Autodesk Inventor part; units mm, degrees
(part 3 of 3)
  spline S409 degree 2 poles (72.0814, -54.0962) (72.3533, -53.7947) (73.1591, -53.4733) (73.6237, -53.4733) knots 0 0 0 1 2 2 2
  spline S410 degree 2 poles (73.6237, -53.4733) (73.9994, -53.4733) (74.7014, -53.6859) (74.9733, -53.8243) knots 0 0 0 1 2 2 2
  line L406 (74.9733, -53.8243) -> (74.9733, -54.6894)
  line L407 (74.9733, -54.6894) -> (74.9288, -54.6894)
  spline S411 degree 2 poles (74.9288, -54.6894) (74.8447, -54.6202) (74.5877, -54.4422) (74.4048, -54.3483) knots 0 0 0 1 2 2 2
  spline S412 degree 2 poles (74.4048, -54.3483) (74.2417, -54.2692) (73.8066, -54.1456) (73.6089, -54.1456) knots 0 0 0 1 2 2 2
  spline S413 degree 2 poles (73.6089, -54.1456) (73.0108, -54.1456) (72.2841, -55.0503) (72.2841, -55.8758) knots 0 0 0 1 2 2 2
  spline S414 degree 2 poles (72.2841, -55.8758) (72.2841, -56.6815) (72.9861, -57.5862) (73.6089, -57.5862) knots 0 0 0 1 2 2 2
  spline S415 degree 2 poles (73.6089, -57.5862) (73.9846, -57.5862) (74.6668, -57.2747) (74.9288, -57.0325) knots 0 0 0 1 2 2 2
  line L408 (74.9288, -57.0325) -> (74.9733, -57.0325)
  line L409 (74.9733, -57.0325) -> (74.9733, -57.8976)
  spline S416 degree 2 poles (74.9733, -57.8976) (74.8596, -57.952) (74.5135, -58.1052) (74.3751, -58.1398) knots 0 0 0 1 2 2 2
  spline S417 degree 2 poles (74.3751, -58.1398) (74.1774, -58.1991) (73.866, -58.2584) (73.6237, -58.2584) knots 0 0 0 1 2 2 2
  line L410 (76.4612, -58.1546) -> (75.69, -58.1546)
  line L411 (75.69, -58.1546) -> (75.69, -53.5772)
  line L412 (75.69, -53.5772) -> (76.4612, -53.5772)
  line L413 (76.4612, -53.5772) -> (76.4612, -58.1546)
  line L414 (76.5156, -52.8159) -> (75.6406, -52.8159)
  line L415 (75.6406, -52.8159) -> (75.6406, -52.0151)
  line L416 (75.6406, -52.0151) -> (76.5156, -52.0151)
  line L417 (76.5156, -52.0151) -> (76.5156, -52.8159)
  line L418 (-27.0263, -68.1981) -> (-27.0263, -62.8198)
  line L419 (-27.0263, -62.8198) -> (-29.0728, -62.8198)
  line L420 (-29.0728, -62.8198) -> (-29.0728, -62.0981)
  line L421 (-29.0728, -62.0981) -> (-24.169, -62.0981)
  line L422 (-24.169, -62.0981) -> (-24.169, -62.8198)
  line L423 (-24.169, -62.8198) -> (-26.2156, -62.8198)
  line L424 (-26.2156, -62.8198) -> (-26.2156, -68.1981)
  line L425 (-26.2156, -68.1981) -> (-27.0263, -68.1981)
  line L426 (-21.1833, -64.4462) -> (-21.2229, -64.4462)
  spline S418 degree 2 poles (-21.2229, -64.4462) (-21.3118, -64.4215) (-21.5046, -64.4116) (-21.6381, -64.4116) knots 0 0 0 1 2 2 2
  spline S419 degree 2 poles (-21.6381, -64.4116) (-21.9495, -64.4116) (-22.5625, -64.6834) (-22.8393, -64.9504) knots 0 0 0 1 2 2 2
  line L427 (-22.8393, -64.9504) -> (-22.8393, -68.1981)
  line L428 (-22.8393, -68.1981) -> (-23.6105, -68.1981)
  line L429 (-23.6105, -68.1981) -> (-23.6105, -63.6206)
  line L430 (-23.6105, -63.6206) -> (-22.8393, -63.6206)
  line L431 (-22.8393, -63.6206) -> (-22.8393, -64.3028)
  spline S420 degree 2 poles (-22.8393, -64.3028) (-22.4191, -63.9271) (-21.7913, -63.6206) (-21.4947, -63.6206) knots 0 0 0 1 2 2 2
  spline S421 degree 2 poles (-21.4947, -63.6206) (-21.3761, -63.6206) (-21.2575, -63.6305) (-21.1833, -63.6454) knots 0 0 0 1 2 2 2
  line L432 (-21.1833, -63.6454) -> (-21.1833, -64.4462)
  line L433 (-19.7992, -68.1981) -> (-20.5703, -68.1981)
  line L434 (-20.5703, -68.1981) -> (-20.5703, -63.6206)
  line L435 (-20.5703, -63.6206) -> (-19.7992, -63.6206)
  line L436 (-19.7992, -63.6206) -> (-19.7992, -68.1981)
  line L437 (-19.7448, -62.8594) -> (-20.6198, -62.8594)
  line L438 (-20.6198, -62.8594) -> (-20.6198, -62.0586)
  line L439 (-20.6198, -62.0586) -> (-19.7448, -62.0586)
  line L440 (-19.7448, -62.0586) -> (-19.7448, -62.8594)
  spline S422 degree 2 poles (-16.68, -68.3019) (-17.7774, -68.3019) (-18.9836, -67.0711) (-18.9836, -65.9341) knots 0 0 0 1 2 2 2
  spline S423 degree 2 poles (-18.9836, -65.9341) (-18.9836, -64.8169) (-17.812, -63.4921) (-16.8678, -63.4921) knots 0 0 0 1 2 2 2
  spline S424 degree 2 poles (-16.8678, -63.4921) (-16.4427, -63.4921) (-15.7853, -63.7393) (-15.543, -64.0013) knots 0 0 0 1 2 2 2
  spline S425 degree 2 poles (-15.543, -64.0013) (-15.2959, -64.2633) (-15.0339, -65.0196) (-15.0339, -65.5683) knots 0 0 0 1 2 2 2
  line L441 (-15.0339, -65.5683) -> (-15.0339, -65.9885)
  line L442 (-15.0339, -65.9885) -> (-18.2025, -65.9885)
  spline S426 degree 2 poles (-18.2025, -65.9885) (-18.2025, -66.7843) (-17.4017, -67.6296) (-16.6899, -67.6296) knots 0 0 0 1 2 2 2
  spline S427 degree 2 poles (-16.6899, -67.6296) (-16.4378, -67.6296) (-15.9484, -67.5159) (-15.7507, -67.427) knots 0 0 0 1 2 2 2
  spline S428 degree 2 poles (-15.7507, -67.427) (-15.543, -67.3281) (-15.2563, -67.1551) (-15.1624, -67.076) knots 0 0 0 1 2 2 2
  line L443 (-15.1624, -67.076) -> (-15.1179, -67.076)
  line L444 (-15.1179, -67.076) -> (-15.1179, -67.9164)
  spline S429 degree 2 poles (-15.1179, -67.9164) (-15.2514, -67.9707) (-15.6567, -68.1289) (-15.8149, -68.1734) knots 0 0 0 1 2 2 2
  spline S430 degree 2 poles (-15.8149, -68.1734) (-16.0374, -68.2377) (-16.4032, -68.3019) (-16.68, -68.3019) knots 0 0 0 1 2 2 2
  spline S431 degree 2 poles (-15.7853, -65.4002) (-15.7951, -65.0888) (-15.9237, -64.634) (-16.0472, -64.4808) knots 0 0 0 1 2 2 2
  spline S432 degree 2 poles (-16.0472, -64.4808) (-16.1807, -64.3078) (-16.6009, -64.1249) (-16.9123, -64.1249) knots 0 0 0 1 2 2 2
  spline S433 degree 2 poles (-16.9123, -64.1249) (-17.2188, -64.1249) (-17.6489, -64.3078) (-17.8268, -64.4857) knots 0 0 0 1 2 2 2
  spline S434 degree 2 poles (-17.8268, -64.4857) (-17.9998, -64.6686) (-18.1778, -65.1086) (-18.2025, -65.4002) knots 0 0 0 1 2 2 2
  line L445 (-18.2025, -65.4002) -> (-15.7853, -65.4002)
  line L446 (-10.6591, -68.1981) -> (-11.4302, -68.1981)
  line L447 (-11.4302, -68.1981) -> (-11.4302, -65.5881)
  spline S435 degree 2 poles (-11.4302, -65.5881) (-11.4302, -65.2717) (-11.4895, -64.7279) (-11.5785, -64.5648) knots 0 0 0 1 2 2 2
  spline S436 degree 2 poles (-11.5785, -64.5648) (-11.6724, -64.3918) (-12.0086, -64.2237) (-12.2953, -64.2237) knots 0 0 0 1 2 2 2
  spline S437 degree 2 poles (-12.2953, -64.2237) (-12.582, -64.2237) (-13.19, -64.5302) (-13.4817, -64.7774) knots 0 0 0 1 2 2 2
  line L448 (-13.4817, -64.7774) -> (-13.4817, -68.1981)
  line L449 (-13.4817, -68.1981) -> (-14.2528, -68.1981)
  line L450 (-14.2528, -68.1981) -> (-14.2528, -63.6206)
  line L451 (-14.2528, -63.6206) -> (-13.4817, -63.6206)
  line L452 (-13.4817, -63.6206) -> (-13.4817, -64.1298)
  spline S438 degree 2 poles (-13.4817, -64.1298) (-13.1357, -63.8184) (-12.4683, -63.4921) (-12.0926, -63.4921) knots 0 0 0 1 2 2 2
  spline S439 degree 2 poles (-12.0926, -63.4921) (-11.4203, -63.4921) (-10.6591, -64.3819) (-10.6591, -65.2272) knots 0 0 0 1 2 2 2
  line L453 (-10.6591, -65.2272) -> (-10.6591, -68.1981)
  line L454 (-5.9827, -68.1981) -> (-6.7539, -68.1981)
  line L455 (-6.7539, -68.1981) -> (-6.7539, -65.5881)
  spline S440 degree 2 poles (-6.7539, -65.5881) (-6.7539, -65.2717) (-6.8132, -64.7279) (-6.9022, -64.5648) knots 0 0 0 1 2 2 2
  spline S441 degree 2 poles (-6.9022, -64.5648) (-6.9961, -64.3918) (-7.3323, -64.2237) (-7.619, -64.2237) knots 0 0 0 1 2 2 2
  spline S442 degree 2 poles (-7.619, -64.2237) (-7.9057, -64.2237) (-8.5137, -64.5302) (-8.8054, -64.7774) knots 0 0 0 1 2 2 2
  line L456 (-8.8054, -64.7774) -> (-8.8054, -68.1981)
  line L457 (-8.8054, -68.1981) -> (-9.5765, -68.1981)
  line L458 (-9.5765, -68.1981) -> (-9.5765, -63.6206)
  line L459 (-9.5765, -63.6206) -> (-8.8054, -63.6206)
  line L460 (-8.8054, -63.6206) -> (-8.8054, -64.1298)
  spline S443 degree 2 poles (-8.8054, -64.1298) (-8.4593, -63.8184) (-7.792, -63.4921) (-7.4163, -63.4921) knots 0 0 0 1 2 2 2
  spline S444 degree 2 poles (-7.4163, -63.4921) (-6.744, -63.4921) (-5.9827, -64.3819) (-5.9827, -65.2272) knots 0 0 0 1 2 2 2
  line L461 (-5.9827, -65.2272) -> (-5.9827, -68.1981)
  spline S445 degree 2 poles (-2.3494, -67.7137) (-2.4434, -67.7829) (-2.7597, -68.03) (-2.908, -68.1042) knots 0 0 0 1 2 2 2
  spline S446 degree 2 poles (-2.908, -68.1042) (-3.1107, -68.2129) (-3.4913, -68.3266) (-3.8374, -68.3266) knots 0 0 0 1 2 2 2
  spline S447 degree 2 poles (-3.8374, -68.3266) (-4.1191, -68.3266) (-4.6283, -68.1141) (-4.8211, -67.9213) knots 0 0 0 1 2 2 2
  spline S448 degree 2 poles (-4.8211, -67.9213) (-5.004, -67.7334) (-5.2264, -67.1798) (-5.2264, -66.8733) knots 0 0 0 1 2 2 2
  spline S449 degree 2 poles (-5.2264, -66.8733) (-5.2264, -66.3988) (-4.826, -65.7265) (-4.391, -65.5337) knots 0 0 0 1 2 2 2
  spline S450 degree 2 poles (-4.391, -65.5337) (-4.0054, -65.3557) (-2.9575, -65.2223) (-2.3494, -65.1877) knots 0 0 0 1 2 2 2
  line L462 (-2.3494, -65.1877) -> (-2.3494, -65.0394)
  spline S451 degree 2 poles (-2.3494, -65.0394) (-2.3494, -64.7724) (-2.5126, -64.4412) (-2.6609, -64.3473) knots 0 0 0 1 2 2 2
  spline S452 degree 2 poles (-2.6609, -64.3473) (-2.8092, -64.2534) (-3.2343, -64.1941) (-3.4617, -64.1941) knots 0 0 0 1 2 2 2
  spline S453 degree 2 poles (-3.4617, -64.1941) (-3.7286, -64.1941) (-4.4503, -64.3522) (-4.8112, -64.5055) knots 0 0 0 1 2 2 2
  line L463 (-4.8112, -64.5055) -> (-4.8557, -64.5055)
  line L464 (-4.8557, -64.5055) -> (-4.8557, -63.7195)
  spline S454 degree 2 poles (-4.8557, -63.7195) (-4.6431, -63.6602) (-3.8472, -63.5119) (-3.4567, -63.5119) knots 0 0 0 1 2 2 2
  spline S455 degree 2 poles (-3.4567, -63.5119) (-2.9822, -63.5119) (-2.3346, -63.6602) (-2.0776, -63.853) knots 0 0 0 1 2 2 2
  spline S456 degree 2 poles (-2.0776, -63.853) (-1.8254, -64.0408) (-1.5783, -64.639) (-1.5783, -65.069) knots 0 0 0 1 2 2 2
  line L465 (-1.5783, -65.069) -> (-1.5783, -68.1981)
  line L466 (-1.5783, -68.1981) -> (-2.3494, -68.1981)
  line L467 (-2.3494, -68.1981) -> (-2.3494, -67.7137)
  line L468 (-2.3494, -67.0711) -> (-2.3494, -65.8006)
  spline S457 degree 2 poles (-2.3494, -65.8006) (-2.6263, -65.8253) (-3.4617, -65.9094) (-3.7237, -65.9885) knots 0 0 0 1 2 2 2
  spline S458 degree 2 poles (-3.7237, -65.9885) (-4.0301, -66.0824) (-4.4306, -66.4729) (-4.4306, -66.8189) knots 0 0 0 1 2 2 2
  spline S459 degree 2 poles (-4.4306, -66.8189) (-4.4306, -67.2144) (-3.9857, -67.6148) (-3.5605, -67.6148) knots 0 0 0 1 2 2 2
  spline S460 degree 2 poles (-3.5605, -67.6148) (-3.1997, -67.6148) (-2.6065, -67.3034) (-2.3494, -67.0711) knots 0 0 0 1 2 2 2
  line L469 (0.2903, -68.1981) -> (-0.4809, -68.1981)
  line L470 (-0.4809, -68.1981) -> (-0.4809, -61.8262)
  line L471 (-0.4809, -61.8262) -> (0.2903, -61.8262)
  line L472 (0.2903, -61.8262) -> (0.2903, -68.1981)
  spline S461 degree 2 poles (3.4095, -68.3019) (2.3121, -68.3019) (1.1059, -67.0711) (1.1059, -65.9341) knots 0 0 0 1 2 2 2
  spline S462 degree 2 poles (1.1059, -65.9341) (1.1059, -64.8169) (2.2775, -63.4921) (3.2216, -63.4921) knots 0 0 0 1 2 2 2
  spline S463 degree 2 poles (3.2216, -63.4921) (3.6468, -63.4921) (4.3042, -63.7393) (4.5464, -64.0013) knots 0 0 0 1 2 2 2
  spline S464 degree 2 poles (4.5464, -64.0013) (4.7936, -64.2633) (5.0556, -65.0196) (5.0556, -65.5683) knots 0 0 0 1 2 2 2
  line L473 (5.0556, -65.5683) -> (5.0556, -65.9885)
  line L474 (5.0556, -65.9885) -> (1.887, -65.9885)
  spline S465 degree 2 poles (1.887, -65.9885) (1.887, -66.7843) (2.6878, -67.6296) (3.3996, -67.6296) knots 0 0 0 1 2 2 2
  spline S466 degree 2 poles (3.3996, -67.6296) (3.6517, -67.6296) (4.1411, -67.5159) (4.3388, -67.427) knots 0 0 0 1 2 2 2
  spline S467 degree 2 poles (4.3388, -67.427) (4.5464, -67.3281) (4.8331, -67.1551) (4.9271, -67.076) knots 0 0 0 1 2 2 2
  line L475 (4.9271, -67.076) -> (4.9716, -67.076)
  line L476 (4.9716, -67.076) -> (4.9716, -67.9164)
  spline S468 degree 2 poles (4.9716, -67.9164) (4.8381, -67.9707) (4.4327, -68.1289) (4.2746, -68.1734) knots 0 0 0 1 2 2 2
  spline S469 degree 2 poles (4.2746, -68.1734) (4.0521, -68.2377) (3.6863, -68.3019) (3.4095, -68.3019) knots 0 0 0 1 2 2 2
  spline S470 degree 2 poles (4.3042, -65.4002) (4.2943, -65.0888) (4.1658, -64.634) (4.0422, -64.4808) knots 0 0 0 1 2 2 2
  spline S471 degree 2 poles (4.0422, -64.4808) (3.9087, -64.3078) (3.4886, -64.1249) (3.1771, -64.1249) knots 0 0 0 1 2 2 2
  spline S472 degree 2 poles (3.1771, -64.1249) (2.8707, -64.1249) (2.4406, -64.3078) (2.2626, -64.4857) knots 0 0 0 1 2 2 2
  spline S473 degree 2 poles (2.2626, -64.4857) (2.0896, -64.6686) (1.9117, -65.1086) (1.887, -65.4002) knots 0 0 0 1 2 2 2
  line L477 (1.887, -65.4002) -> (4.3042, -65.4002)
  line L478 (12.1047, -68.1981) -> (8.3429, -68.1981)
  line L479 (8.3429, -68.1981) -> (8.3429, -67.333)
  spline S474 degree 2 poles (8.3429, -67.333) (8.7482, -66.9524) (9.4699, -66.2455) (9.816, -65.8649) knots 0 0 0 1 2 2 2
  spline S475 degree 2 poles (9.816, -65.8649) (10.513, -65.0987) (11.0221, -64.1792) (11.0221, -63.6899) knots 0 0 0 1 2 2 2
  spline S476 degree 2 poles (11.0221, -63.6899) (11.0221, -63.4328) (10.8639, -63.0472) (10.7206, -62.9236) knots 0 0 0 1 2 2 2
  spline S477 degree 2 poles (10.7206, -62.9236) (10.5772, -62.8001) (10.2015, -62.6765) (9.9741, -62.6765) knots 0 0 0 1 2 2 2
  spline S478 degree 2 poles (9.9741, -62.6765) (9.7566, -62.6765) (9.3117, -62.7852) (9.1091, -62.8693) knots 0 0 0 1 2 2 2
  spline S479 degree 2 poles (9.1091, -62.8693) (8.9361, -62.9385) (8.6147, -63.1362) (8.5159, -63.2054) knots 0 0 0 1 2 2 2
  line L480 (8.5159, -63.2054) -> (8.4714, -63.2054)
  line L481 (8.4714, -63.2054) -> (8.4714, -62.3354)
  spline S480 degree 2 poles (8.4714, -62.3354) (8.7235, -62.2118) (9.6281, -61.9696) (10.0335, -61.9696) knots 0 0 0 1 2 2 2
  spline S481 degree 2 poles (10.0335, -61.9696) (10.8887, -61.9696) (11.8526, -62.8742) (11.8526, -63.6454) knots 0 0 0 1 2 2 2
  spline S482 degree 2 poles (11.8526, -63.6454) (11.8526, -64.0062) (11.6845, -64.6093) (11.5362, -64.8664) knots 0 0 0 1 2 2 2
  spline S483 degree 2 poles (11.5362, -64.8664) (11.3879, -65.1333) (10.9579, -65.6573) (10.7206, -65.9094) knots 0 0 0 1 2 2 2
  spline S484 degree 2 poles (10.7206, -65.9094) (10.335, -66.3296) (9.3908, -67.2292) (9.1091, -67.4912) knots 0 0 0 1 2 2 2
  line L482 (9.1091, -67.4912) -> (12.1047, -67.4912)
  line L483 (12.1047, -67.4912) -> (12.1047, -68.1981)
  spline S485 degree 2 poles (16.7168, -65.1481) (16.7168, -66.7893) (15.7627, -68.3266) (14.7691, -68.3266) knots 0 0 0 1 2 2 2
  spline S486 degree 2 poles (14.7691, -68.3266) (13.7607, -68.3266) (12.8165, -66.7596) (12.8165, -65.1531) knots 0 0 0 1 2 2 2
  spline S487 degree 2 poles (12.8165, -65.1531) (12.8165, -63.502) (13.7706, -61.9745) (14.7691, -61.9745) knots 0 0 0 1 2 2 2
  spline S488 degree 2 poles (14.7691, -61.9745) (15.7726, -61.9745) (16.7168, -63.5564) (16.7168, -65.1481) knots 0 0 0 1 2 2 2
  spline S489 degree 2 poles (15.6688, -67.0068) (15.7874, -66.7052) (15.8863, -65.7759) (15.8863, -65.1481) knots 0 0 0 1 2 2 2
  spline S490 degree 2 poles (15.8863, -65.1481) (15.8863, -64.5203) (15.7874, -63.5959) (15.6639, -63.2845) knots 0 0 0 1 2 2 2
  spline S491 degree 2 poles (15.6639, -63.2845) (15.5403, -62.9731) (15.1102, -62.6518) (14.7691, -62.6518) knots 0 0 0 1 2 2 2
  spline S492 degree 2 poles (14.7691, -62.6518) (14.428, -62.6518) (13.9881, -62.9731) (13.8596, -63.2944) knots 0 0 0 1 2 2 2
  spline S493 degree 2 poles (13.8596, -63.2944) (13.736, -63.6058) (13.647, -64.5549) (13.647, -65.1531) knots 0 0 0 1 2 2 2
  spline S494 degree 2 poles (13.647, -65.1531) (13.647, -65.7957) (13.7261, -66.6558) (13.8546, -66.992) knots 0 0 0 1 2 2 2
  spline S495 degree 2 poles (13.8546, -66.992) (13.9733, -67.3083) (14.4132, -67.6494) (14.7691, -67.6494) knots 0 0 0 1 2 2 2
  spline S496 degree 2 poles (14.7691, -67.6494) (15.1053, -67.6494) (15.5452, -67.3281) (15.6688, -67.0068) knots 0 0 0 1 2 2 2
  line L484 (20.9532, -68.1981) -> (17.9773, -68.1981)
  line L485 (17.9773, -68.1981) -> (17.9773, -67.5753)
  line L486 (17.9773, -67.5753) -> (19.0846, -67.5753)
  line L487 (19.0846, -67.5753) -> (19.0846, -63.4872)
  line L488 (19.0846, -63.4872) -> (17.9773, -63.4872)
  line L489 (17.9773, -63.4872) -> (17.9773, -62.9286)
  spline S497 degree 2 poles (17.9773, -62.9286) (18.6051, -62.9286) (19.1983, -62.5727) (19.2378, -62.0783) knots 0 0 0 1 2 2 2
  line L490 (19.2378, -62.0783) -> (19.8706, -62.0783)
  line L491 (19.8706, -62.0783) -> (19.8706, -67.5753)
  line L492 (19.8706, -67.5753) -> (20.9532, -67.5753)
  line L493 (20.9532, -67.5753) -> (20.9532, -68.1981)
  spline S498 degree 2 poles (23.9191, -68.3365) (23.4643, -68.3365) (22.7179, -68.0646) (22.4559, -67.8125) knots 0 0 0 1 2 2 2
  spline S499 degree 2 poles (22.4559, -67.8125) (22.1989, -67.5654) (21.9319, -66.8931) (21.9319, -66.5125) knots 0 0 0 1 2 2 2
  spline S500 degree 2 poles (21.9319, -66.5125) (21.9319, -66.0181) (22.4609, -65.1877) (22.9651, -64.9405) knots 0 0 0 1 2 2 2
  line L494 (22.9651, -64.9405) -> (22.9651, -64.9158)
  spline S501 degree 2 poles (22.9651, -64.9158) (22.5152, -64.6538) (22.0802, -64.0309) (22.0802, -63.5663) knots 0 0 0 1 2 2 2
  spline S502 degree 2 poles (22.0802, -63.5663) (22.0802, -62.8792) (23.1183, -61.9597) (23.9191, -61.9597) knots 0 0 0 1 2 2 2
  spline S503 degree 2 poles (23.9191, -61.9597) (24.7496, -61.9597) (25.7531, -62.8297) (25.7531, -63.5119) knots 0 0 0 1 2 2 2
  spline S504 degree 2 poles (25.7531, -63.5119) (25.7531, -63.9222) (25.2736, -64.723) (24.8237, -64.9504) knots 0 0 0 1 2 2 2
  line L495 (24.8237, -64.9504) -> (24.8237, -64.9751)
  spline S505 degree 2 poles (24.8237, -64.9751) (25.3576, -65.2223) (25.9063, -65.9341) (25.9063, -66.4976) knots 0 0 0 1 2 2 2
  spline S506 degree 2 poles (25.9063, -66.4976) (25.9063, -67.2787) (24.7694, -68.3365) (23.9191, -68.3365) knots 0 0 0 1 2 2 2
  spline S507 degree 2 poles (25.066, -66.5767) (25.066, -66.201) (24.7694, -65.7561) (24.3492, -65.5287) knots 0 0 0 1 2 2 2
  spline S508 degree 2 poles (24.3492, -65.5287) (24.2108, -65.4497) (23.7461, -65.2668) (23.4545, -65.1481) knots 0 0 0 1 2 2 2
  spline S509 degree 2 poles (23.4545, -65.1481) (23.1183, -65.3706) (22.7575, -66.033) (22.7575, -66.4531) knots 0 0 0 1 2 2 2
  spline S510 degree 2 poles (22.7575, -66.4531) (22.7575, -67.0068) (23.4248, -67.7285) (23.929, -67.7285) knots 0 0 0 1 2 2 2
  spline S511 degree 2 poles (23.929, -67.7285) (24.4431, -67.7285) (25.066, -67.1106) (25.066, -66.5767) knots 0 0 0 1 2 2 2
  spline S512 degree 2 poles (24.9523, -63.5218) (24.9523, -63.1115) (24.4036, -62.5628) (23.9142, -62.5628) knots 0 0 0 1 2 2 2
  spline S513 degree 2 poles (23.9142, -62.5628) (23.4693, -62.5628) (22.9008, -63.0522) (22.9008, -63.4723) knots 0 0 0 1 2 2 2
  spline S514 degree 2 poles (22.9008, -63.4723) (22.9008, -63.7739) (23.1925, -64.1941) (23.4841, -64.3621) knots 0 0 0 1 2 2 2
  spline S515 degree 2 poles (23.4841, -64.3621) (23.6077, -64.4313) (24.1317, -64.6736) (24.3442, -64.7428) knots 0 0 0 1 2 2 2
  spline S516 degree 2 poles (24.3442, -64.7428) (24.7002, -64.4709) (24.9523, -63.8925) (24.9523, -63.5218) knots 0 0 0 1 2 2 2
  line L496 (29.1887, -61.8262) -> (26.8011, -69.5229)
  line L497 (26.8011, -69.5229) -> (26.109, -69.5229)
  line L498 (26.109, -69.5229) -> (28.4867, -61.8262)
  line L499 (28.4867, -61.8262) -> (29.1887, -61.8262)
  line L500 (33.3163, -68.1981) -> (30.3404, -68.1981)
  line L501 (30.3404, -68.1981) -> (30.3404, -67.5753)
  line L502 (30.3404, -67.5753) -> (31.4477, -67.5753)
  line L503 (31.4477, -67.5753) -> (31.4477, -63.4872)
  line L504 (31.4477, -63.4872) -> (30.3404, -63.4872)
  line L505 (30.3404, -63.4872) -> (30.3404, -62.9286)
  spline S517 degree 2 poles (30.3404, -62.9286) (30.9682, -62.9286) (31.5614, -62.5727) (31.601, -62.0783) knots 0 0 0 1 2 2 2
  line L506 (31.601, -62.0783) -> (32.2337, -62.0783)
  line L507 (32.2337, -62.0783) -> (32.2337, -67.5753)
  line L508 (32.2337, -67.5753) -> (33.3163, -67.5753)
  line L509 (33.3163, -67.5753) -> (33.3163, -68.1981)
  spline S518 degree 2 poles (34.2703, -64.0804) (34.2703, -63.6108) (34.5768, -62.8297) (34.8438, -62.548) knots 0 0 0 1 2 2 2
  spline S519 degree 2 poles (34.8438, -62.548) (35.0959, -62.2761) (35.8324, -61.9745) (36.2081, -61.9745) knots 0 0 0 1 2 2 2
  spline S520 degree 2 poles (36.2081, -61.9745) (36.6283, -61.9745) (37.3105, -62.2563) (37.5626, -62.5232) knots 0 0 0 1 2 2 2
  spline S521 degree 2 poles (37.5626, -62.5232) (37.8789, -62.8594) (38.225, -63.9469) (38.225, -64.7823) knots 0 0 0 1 2 2 2
  spline S522 degree 2 poles (38.225, -64.7823) (38.225, -65.5386) (37.8839, -66.8931) (37.5527, -67.3429) knots 0 0 0 1 2 2 2
  spline S523 degree 2 poles (37.5527, -67.3429) (37.2017, -67.8175) (36.213, -68.3168) (35.4913, -68.3168) knots 0 0 0 1 2 2 2
  spline S524 degree 2 poles (35.4913, -68.3168) (35.3282, -68.3168) (34.9575, -68.2822) (34.7993, -68.2327) knots 0 0 0 1 2 2 2
  line L510 (34.7993, -68.2327) -> (34.7993, -67.4467)
  line L511 (34.7993, -67.4467) -> (34.8388, -67.4467)
  spline S525 degree 2 poles (34.8388, -67.4467) (34.9426, -67.5061) (35.3776, -67.6099) (35.6001, -67.6099) knots 0 0 0 1 2 2 2
  spline S526 degree 2 poles (35.6001, -67.6099) (36.4009, -67.6099) (37.3154, -66.552) (37.3797, -65.5732) knots 0 0 0 1 2 2 2
  spline S527 degree 2 poles (37.3797, -65.5732) (37.0534, -65.7957) (36.4602, -65.9984) (36.1092, -65.9984) knots 0 0 0 1 2 2 2
  spline S528 degree 2 poles (36.1092, -65.9984) (35.7731, -65.9984) (35.2145, -65.8501) (34.9327, -65.6375) knots 0 0 0 1 2 2 2
  spline S529 degree 2 poles (34.9327, -65.6375) (34.6065, -65.3854) (34.2703, -64.6192) (34.2703, -64.0804) knots 0 0 0 1 2 2 2
  spline S530 degree 2 poles (37.3994, -64.5994) (37.3994, -63.9815) (37.172, -63.2005) (36.9694, -62.9879) knots 0 0 0 1 2 2 2
  spline S531 degree 2 poles (36.9694, -62.9879) (36.7914, -62.7902) (36.4207, -62.6419) (36.2032, -62.6419) knots 0 0 0 1 2 2 2
  spline S532 degree 2 poles (36.2032, -62.6419) (35.6989, -62.6419) (35.1008, -63.3636) (35.1008, -64.0458) knots 0 0 0 1 2 2 2
  spline S533 degree 2 poles (35.1008, -64.0458) (35.1008, -64.4313) (35.2985, -64.9306) (35.516, -65.1086) knots 0 0 0 1 2 2 2
  spline S534 degree 2 poles (35.516, -65.1086) (35.6742, -65.2371) (36.0647, -65.3211) (36.2921, -65.3211) knots 0 0 0 1 2 2 2
  spline S535 degree 2 poles (36.2921, -65.3211) (36.5541, -65.3211) (37.1572, -65.1382) (37.3846, -64.985) knots 0 0 0 1 2 2 2
  spline S536 degree 2 poles (37.3846, -64.985) (37.3895, -64.9257) (37.3994, -64.723) (37.3994, -64.5994) knots 0 0 0 1 2 2 2
  point P0 (0, 0)
  constraints: 5 other
extrude "Estrusione5" cut sketch "Schizzo6" against normal blind 1
